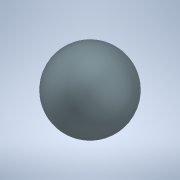
# Autodesk Inventor part: bump bond
Saved by Autodesk Inventor 2022 (Build 260153000, 153)
## iProperties
Created: 2022-02-01
Part Number: bump bond
Material: Lead
Document SubType Name: Modeling
Designer: Caleb
Density: 11.34 g/cm^3
Appearance: Lead
Author: Caleb
Autodesk Inventor part; units mm, degrees
ref_plane "YZ Plane" through (0, 0, 0) normal (1, 0, 0) x (0, 1, 0)
ref_plane "XZ Plane" through (0, 0, 0) normal (0, 1, 0) x (-1, 0, 0)
ref_plane "XY Plane" through (0, 0, 0) normal (0, 0, 1) x (1, 0, 0)
sketch "Sketch1" plane through (0, 0, 0) normal (0, 1, 0) x (-1, 0, 0)
  arc A0 (0, 0.04) -> (0, -0.04) centre (0, 0) ccw
  line L0 (0, 0) -> (0, -0.04) construction
  line L1 (0, 0) -> (0.04, 0) construction
  line L2 (0, 0) -> (0, 0.04) construction
  line L3 (0, 0.04) -> (0, -0.04)
  dimension "d5" = 0.04
  dimension "d6" = 90
  dimension "d7" = 180
  constraints: 8 end point, 2 point on circle, 1 centre point, 1 horizontal, 1 perpendicular
  measures "d5" radius of A0
  measures "d6" angle of L0 L1
  measures "d7" angle of L0 L2
revolve "Revolution1" add sketch "Sketch1" angle 360 about axis through (0, 0, 0) along (0, 0, -1)
body "Solid1"
